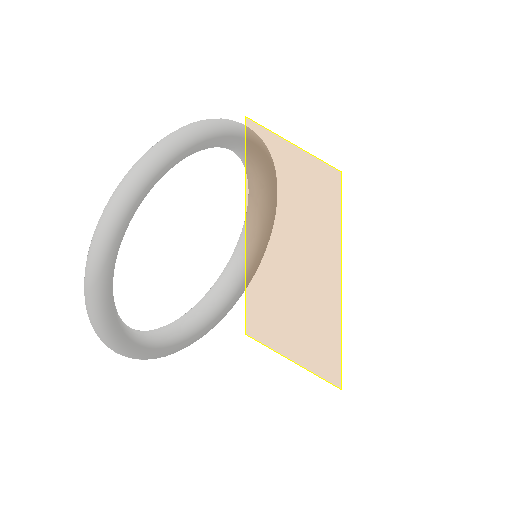
# Autodesk Inventor part: 00_0-ring
Saved by Autodesk Inventor 2023 (Build 270158000, 158)
## iProperties
Created: 2021-11-24
Part Number: 00_0-ring
Material: Generisch
Document SubType Name: Modeling
Designer: Muriel
Density: 1 g/cm^3
Appearance: Vorgabe
Author: Muriel
Autodesk Inventor part; units mm, degrees
ref_plane "YZ Plane" through (0, 0, 0) normal (1, 0, 0) x (0, 1, 0)
ref_plane "XZ Plane" through (0, 0, 0) normal (0, 1, 0) x (-1, 0, 0)
ref_plane "XY Plane" through (0, 0, 0) normal (0, 0, 1) x (1, 0, 0)
ref_plane "Arbeitsebene1" through (11.2054, 6.4475, 348.4816) normal (0, 0, 1) x (1, 0, 0)
sketch "Skizze1" plane through (11.2054, 6.4475, 348.4816) normal (0, 0, 1) x (1, 0, 0)
  circle A0 centre (-15.666, -18.4475) radius 1.5
  line L0 (-18.3582, -6.4475) -> (-10.0133, -6.4475) projected
  point P0 (-11.2054, -6.4475)
  dimension "d0" = 3
  dimension "d1" = 12
  constraints: 1 centre point
  measures "d0" diameter of A0
  measures "d1" vertical distance of A0.centre point (-11.205, -6.448)
revolve "Umdrehung1" add sketch "Skizze1" angle 360 about axis through (-10, 0, 348.4816) along (1, 0, 0)
